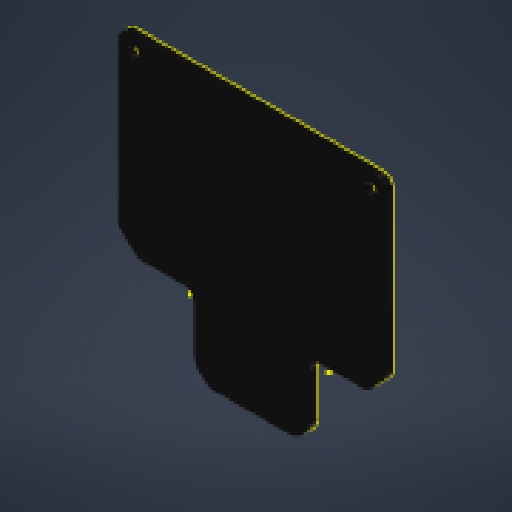
# Autodesk Inventor part: Motor Driver Board
Saved by Autodesk Inventor 2026.1 (Build 301233020, 233B)
## iProperties
Created: 2026-04-03
Part Number: Motor Driver Board
Material: Generic
Document SubType Name: Modeling
Designer: Bahaa
Density: 1 g/cm^3
Appearance: Glossy - Black
Mass: 8.08903 g
Surface Area: 86.5661 cm^2
Volume: 8.08903 cm^3
Author: Bahaa
Autodesk Inventor part; units mm, degrees
ref_plane "YZ Plane" through (0, 0, 0) normal (1, 0, 0) x (0, 1, 0)
ref_plane "XZ Plane" through (0, 0, 0) normal (0, 1, 0) x (-1, 0, 0)
ref_plane "XY Plane" through (0, 0, 0) normal (0, 0, 1) x (1, 0, 0)
sketch "Sketch1" plane through (0, 0, 0) normal (0, 1, 0) x (-1, 0, 0)
  line L0 (35, 25) -> (-35, 25)
  line L1 (-35, 25) -> (-35, -20)
  line L2 (-30, -25) -> (30, -25)
  line L3 (35, -20) -> (35, 25)
  line L4 (35, 25) -> (-35, -25) construction
  line L5 (-35, 25) -> (35, -25) construction
  line L6 (35, 25) -> (31, 25)
  line L7 (31, 25) -> (31, 21) construction
  line L8 (31, 21) -> (35, 21) construction
  line L9 (35, 21) -> (35, 25)
  line L10 (0, 25) -> (0, -25) construction
  circle A0 centre (31, 21) radius 1.6
  circle A1 centre (-31, 21) radius 1.6
  line L11 (15, -45) -> (-15, -45)
  line L12 (-15, -45) -> (-15, -5)
  line L13 (-15, -5) -> (15, -5)
  line L14 (15, -5) -> (15, -45)
  line L15 (15, -45) -> (-15, -5) construction
  line L16 (-15, -45) -> (15, -5) construction
  line L17 (27, 17) -> (35, 17) construction
  line L18 (35, 17) -> (35, 25) construction
  line L19 (35, 25) -> (27, 25) construction
  line L20 (27, 25) -> (27, 17) construction
  line L21 (27, 17) -> (35, 25) construction
  line L22 (35, 17) -> (27, 25) construction
  line L23 (-27, 17) -> (-35, 17) construction
  line L24 (-35, 17) -> (-35, 25) construction
  line L25 (-35, 25) -> (-27, 25) construction
  line L26 (-27, 25) -> (-27, 17) construction
  line L27 (-27, 17) -> (-35, 25) construction
  line L28 (-35, 17) -> (-27, 25) construction
  line L29 (35, -20) -> (30, -25)
  line L30 (-30, -25) -> (-35, -20)
  point P0 (0, 0)
  point P1 (15, -25)
  point P2 (-15, -25)
  dimension "d0" = 70
  dimension "d1" = 50
  dimension "d11" = 4
  dimension "d12" = 4
  dimension "d13" = 3.2
  dimension "d14" = 30
  dimension "d15" = 40
  dimension "d16" = 5
  dimension "d17" = 5
  dimension "d18" = 5
  dimension "d19" = 5
  constraints: 62 end point, 10 midpoint, 10 parallel, 5 horizontal, 5 perpendicular, 4 point on line, 2 centre point, 2 coincident, 1 symmetric about line, 1 other
  measures "d0" distance of L5.end L4.end
  measures "d1" distance of L4.end L0.end
  measures "d11" distance of L8.end L7.end
  measures "d12" distance of L7.end L6.end
  measures "d13" diameter of A0
  measures "d14" distance between parallel lines of L12 L14
  measures "d15" distance of L11.end L12.end
  measures "d16" distance of L3.start L5.end
  measures "d17" distance of L2.end L5.end
  measures "d18" distance of L2.start L4.end
  measures "d19" distance of L1.end L4.end
extrude "Extrusion1" add sketch "Sketch1" along normal blind 2
fillet "Fillet1" radius 3 8 edges at (-35, 1, 25) (35, 1, 25) (-15, 1, -25) (15, 1, -25) (30, 1, -25) (35, 1, -20) (-35, 1, -20) (-30, 1, -25)
chamfer "Chamfer1" distance 3.5 angle 45 2 edges at (-15, 1, -45) (15, 1, -45)
fillet "Fillet3" radius 4 4 edges at (15, 1, -41.5) (11.5, 1, -45) (-11.5, 1, -45) (-15, 1, -41.5)
sketch "Sketch2" plane through (0, 2, 0) normal (0, 1, 0) x (1, 0, 0)
  arc A0 (-9.8431, 45) -> (-12.6716, 43.8284) centre (-9.8431, 41) ccw projected
  line L0 (-9.8431, 45) -> (9.8431, 45) projected
  arc A1 (12.6716, 43.8284) -> (9.8431, 45) centre (9.8431, 41) ccw projected
  line L1 (12.6716, 43.8284) -> (13.8284, 42.6716) projected
  arc A2 (15, 39.8431) -> (13.8284, 42.6716) centre (11, 39.8431) ccw projected
  line L2 (15, 39.8431) -> (15, 28) projected
  arc A3 (15, 28) -> (18, 25) centre (18, 28) ccw projected
  line L3 (18, 25) -> (28.7574, 25) projected
  arc A4 (30.8787, 24.1213) -> (28.7574, 25) centre (28.7574, 22) ccw projected
  line L4 (30.8787, 24.1213) -> (34.1213, 20.8787) projected
  arc A5 (35, 18.7574) -> (34.1213, 20.8787) centre (32, 18.7574) ccw projected
  line L5 (35, 18.7574) -> (35, -22) projected
  arc A6 (32, -25) -> (35, -22) centre (32, -22) ccw projected
  line L6 (32, -25) -> (-32, -25) projected
  arc A7 (-35, -22) -> (-32, -25) centre (-32, -22) ccw projected
  line L7 (-35, -22) -> (-35, 18.7574) projected
  arc A8 (-34.1213, 20.8787) -> (-35, 18.7574) centre (-32, 18.7574) ccw projected
  line L8 (-34.1213, 20.8787) -> (-30.8787, 24.1213) projected
  arc A9 (-28.7574, 25) -> (-30.8787, 24.1213) centre (-28.7574, 22) ccw projected
  line L9 (-28.7574, 25) -> (-18, 25) projected
  arc A10 (-18, 25) -> (-15, 28) centre (-18, 28) ccw projected
  line L10 (-15, 28) -> (-15, 39.8431) projected
  arc A11 (-13.8284, 42.6716) -> (-15, 39.8431) centre (-11, 39.8431) ccw projected
  line L11 (-13.8284, 42.6716) -> (-12.6716, 43.8284) projected
  circle A12 centre (31, -21) radius 1.6 projected
  circle A13 centre (-31, -21) radius 1.6 projected
  line L12 (-13.31, 26.23) -> (-13.31, 38.93)
  line L13 (-13.31, 38.93) -> (-8.23, 38.93)
  line L14 (-8.23, 38.93) -> (-8.23, 26.23)
  line L15 (-8.23, 26.23) -> (-13.31, 26.23)
  line L16 (-12.14, 37.96) -> (-12.34, 37.96)
  line L17 (-12.34, 37.96) -> (-12.34, 37.36)
  line L18 (-12.34, 37.36) -> (-12.14, 37.36)
  line L19 (-12.14, 37.36) -> (-12.14, 37.41)
  line L20 (-12.14, 37.41) -> (-11.94, 37.41)
  line L21 (-11.94, 37.41) -> (-11.94, 37.36)
  line L22 (-11.94, 37.36) -> (-11.74, 37.36)
  line L23 (-11.74, 37.36) -> (-11.74, 37.96)
  line L24 (-11.74, 37.96) -> (-11.94, 37.96)
  line L25 (-11.94, 37.96) -> (-11.94, 37.91)
  line L26 (-11.94, 37.91) -> (-12.14, 37.91)
  line L27 (-12.14, 37.91) -> (-12.14, 37.96)
  line L28 (-12.14, 35.42) -> (-12.34, 35.42)
  line L29 (-12.34, 35.42) -> (-12.34, 34.82)
  line L30 (-12.34, 34.82) -> (-12.14, 34.82)
  line L31 (-12.14, 34.82) -> (-12.14, 34.87)
  line L32 (-12.14, 34.87) -> (-11.94, 34.87)
  line L33 (-11.94, 34.87) -> (-11.94, 34.82)
  line L34 (-11.94, 34.82) -> (-11.74, 34.82)
  line L35 (-11.74, 34.82) -> (-11.74, 35.42)
  line L36 (-11.74, 35.42) -> (-11.94, 35.42)
  line L37 (-11.94, 35.42) -> (-11.94, 35.37)
  line L38 (-11.94, 35.37) -> (-12.14, 35.37)
  line L39 (-12.14, 35.37) -> (-12.14, 35.42)
  line L40 (-12.14, 32.88) -> (-12.34, 32.88)
  line L41 (-12.34, 32.88) -> (-12.34, 32.28)
  line L42 (-12.34, 32.28) -> (-12.14, 32.28)
  line L43 (-12.14, 32.28) -> (-12.14, 32.33)
  line L44 (-12.14, 32.33) -> (-11.94, 32.33)
  line L45 (-11.94, 32.33) -> (-11.94, 32.28)
  line L46 (-11.94, 32.28) -> (-11.74, 32.28)
  line L47 (-11.74, 32.28) -> (-11.74, 32.88)
  line L48 (-11.74, 32.88) -> (-11.94, 32.88)
  line L49 (-11.94, 32.88) -> (-11.94, 32.83)
  line L50 (-11.94, 32.83) -> (-12.14, 32.83)
  line L51 (-12.14, 32.83) -> (-12.14, 32.88)
  line L52 (-12.14, 30.34) -> (-12.34, 30.34)
  line L53 (-12.34, 30.34) -> (-12.34, 29.74)
  line L54 (-12.34, 29.74) -> (-12.14, 29.74)
  line L55 (-12.14, 29.74) -> (-12.14, 29.79)
  line L56 (-12.14, 29.79) -> (-11.94, 29.79)
  line L57 (-11.94, 29.79) -> (-11.94, 29.74)
  line L58 (-11.94, 29.74) -> (-11.74, 29.74)
  line L59 (-11.74, 29.74) -> (-11.74, 30.34)
  line L60 (-11.74, 30.34) -> (-11.94, 30.34)
  line L61 (-11.94, 30.34) -> (-11.94, 30.29)
  line L62 (-11.94, 30.29) -> (-12.14, 30.29)
  line L63 (-12.14, 30.29) -> (-12.14, 30.34)
  line L64 (-12.14, 27.8) -> (-12.34, 27.8)
  line L65 (-12.34, 27.8) -> (-12.34, 27.2)
  line L66 (-12.34, 27.2) -> (-12.14, 27.2)
  line L67 (-12.14, 27.2) -> (-12.14, 27.25)
  line L68 (-12.14, 27.25) -> (-11.94, 27.25)
  line L69 (-11.94, 27.25) -> (-11.94, 27.2)
  line L70 (-11.94, 27.2) -> (-11.74, 27.2)
  line L71 (-11.74, 27.2) -> (-11.74, 27.8)
  line L72 (-11.74, 27.8) -> (-11.94, 27.8)
  line L73 (-11.94, 27.8) -> (-11.94, 27.75)
  line L74 (-11.94, 27.75) -> (-12.14, 27.75)
  line L75 (-12.14, 27.75) -> (-12.14, 27.8)
  line L76 (-9.4, 37.36) -> (-9.2, 37.36)
  line L77 (-9.2, 37.36) -> (-9.2, 37.96)
  line L78 (-9.2, 37.96) -> (-9.4, 37.96)
  line L79 (-9.4, 37.96) -> (-9.4, 37.91)
  line L80 (-9.4, 37.91) -> (-9.6, 37.91)
  line L81 (-9.6, 37.91) -> (-9.6, 37.96)
  line L82 (-9.6, 37.96) -> (-9.8, 37.96)
  line L83 (-9.8, 37.96) -> (-9.8, 37.36)
  line L84 (-9.8, 37.36) -> (-9.6, 37.36)
  line L85 (-9.6, 37.36) -> (-9.6, 37.41)
  line L86 (-9.6, 37.41) -> (-9.4, 37.41)
  line L87 (-9.4, 37.41) -> (-9.4, 37.36)
  line L88 (-9.4, 34.82) -> (-9.2, 34.82)
  line L89 (-9.2, 34.82) -> (-9.2, 35.42)
  line L90 (-9.2, 35.42) -> (-9.4, 35.42)
  line L91 (-9.4, 35.42) -> (-9.4, 35.37)
  line L92 (-9.4, 35.37) -> (-9.6, 35.37)
  line L93 (-9.6, 35.37) -> (-9.6, 35.42)
  line L94 (-9.6, 35.42) -> (-9.8, 35.42)
  line L95 (-9.8, 35.42) -> (-9.8, 34.82)
  line L96 (-9.8, 34.82) -> (-9.6, 34.82)
  line L97 (-9.6, 34.82) -> (-9.6, 34.87)
  line L98 (-9.6, 34.87) -> (-9.4, 34.87)
  line L99 (-9.4, 34.87) -> (-9.4, 34.82)
  line L100 (-9.4, 32.28) -> (-9.2, 32.28)
  line L101 (-9.2, 32.28) -> (-9.2, 32.88)
  line L102 (-9.2, 32.88) -> (-9.4, 32.88)
  line L103 (-9.4, 32.88) -> (-9.4, 32.83)
  line L104 (-9.4, 32.83) -> (-9.6, 32.83)
  line L105 (-9.6, 32.83) -> (-9.6, 32.88)
  line L106 (-9.6, 32.88) -> (-9.8, 32.88)
  line L107 (-9.8, 32.88) -> (-9.8, 32.28)
  line L108 (-9.8, 32.28) -> (-9.6, 32.28)
  line L109 (-9.6, 32.28) -> (-9.6, 32.33)
  line L110 (-9.6, 32.33) -> (-9.4, 32.33)
  line L111 (-9.4, 32.33) -> (-9.4, 32.28)
  line L112 (-9.4, 29.74) -> (-9.2, 29.74)
  line L113 (-9.2, 29.74) -> (-9.2, 30.34)
  line L114 (-9.2, 30.34) -> (-9.4, 30.34)
  line L115 (-9.4, 30.34) -> (-9.4, 30.29)
  line L116 (-9.4, 30.29) -> (-9.6, 30.29)
  line L117 (-9.6, 30.29) -> (-9.6, 30.34)
  line L118 (-9.6, 30.34) -> (-9.8, 30.34)
  line L119 (-9.8, 30.34) -> (-9.8, 29.74)
  line L120 (-9.8, 29.74) -> (-9.6, 29.74)
  line L121 (-9.6, 29.74) -> (-9.6, 29.79)
  line L122 (-9.6, 29.79) -> (-9.4, 29.79)
  line L123 (-9.4, 29.79) -> (-9.4, 29.74)
  line L124 (-9.4, 27.2) -> (-9.2, 27.2)
  line L125 (-9.2, 27.2) -> (-9.2, 27.8)
  line L126 (-9.2, 27.8) -> (-9.4, 27.8)
  line L127 (-9.4, 27.8) -> (-9.4, 27.75)
  line L128 (-9.4, 27.75) -> (-9.6, 27.75)
  line L129 (-9.6, 27.75) -> (-9.6, 27.8)
  line L130 (-9.6, 27.8) -> (-9.8, 27.8)
  line L131 (-9.8, 27.8) -> (-9.8, 27.2)
  line L132 (-9.8, 27.2) -> (-9.6, 27.2)
  line L133 (-9.6, 27.2) -> (-9.6, 27.25)
  line L134 (-9.6, 27.25) -> (-9.4, 27.25)
  line L135 (-9.4, 27.25) -> (-9.4, 27.2)
  line L136 (8.23, 26.23) -> (8.23, 38.93)
  line L137 (8.23, 38.93) -> (13.31, 38.93)
  line L138 (13.31, 38.93) -> (13.31, 26.23)
  line L139 (13.31, 26.23) -> (8.23, 26.23)
  line L140 (9.4, 37.96) -> (9.2, 37.96)
  line L141 (9.2, 37.96) -> (9.2, 37.36)
  line L142 (9.2, 37.36) -> (9.4, 37.36)
  line L143 (9.4, 37.36) -> (9.4, 37.41)
  line L144 (9.4, 37.41) -> (9.6, 37.41)
  line L145 (9.6, 37.41) -> (9.6, 37.36)
  line L146 (9.6, 37.36) -> (9.8, 37.36)
  line L147 (9.8, 37.36) -> (9.8, 37.96)
  line L148 (9.8, 37.96) -> (9.6, 37.96)
  line L149 (9.6, 37.96) -> (9.6, 37.91)
  line L150 (9.6, 37.91) -> (9.4, 37.91)
  line L151 (9.4, 37.91) -> (9.4, 37.96)
  line L152 (9.4, 35.42) -> (9.2, 35.42)
  line L153 (9.2, 35.42) -> (9.2, 34.82)
  line L154 (9.2, 34.82) -> (9.4, 34.82)
  line L155 (9.4, 34.82) -> (9.4, 34.87)
  line L156 (9.4, 34.87) -> (9.6, 34.87)
  line L157 (9.6, 34.87) -> (9.6, 34.82)
  line L158 (9.6, 34.82) -> (9.8, 34.82)
  line L159 (9.8, 34.82) -> (9.8, 35.42)
  line L160 (9.8, 35.42) -> (9.6, 35.42)
  line L161 (9.6, 35.42) -> (9.6, 35.37)
  line L162 (9.6, 35.37) -> (9.4, 35.37)
  line L163 (9.4, 35.37) -> (9.4, 35.42)
  line L164 (9.4, 32.88) -> (9.2, 32.88)
  line L165 (9.2, 32.88) -> (9.2, 32.28)
  line L166 (9.2, 32.28) -> (9.4, 32.28)
  line L167 (9.4, 32.28) -> (9.4, 32.33)
  line L168 (9.4, 32.33) -> (9.6, 32.33)
  line L169 (9.6, 32.33) -> (9.6, 32.28)
  line L170 (9.6, 32.28) -> (9.8, 32.28)
  line L171 (9.8, 32.28) -> (9.8, 32.88)
  line L172 (9.8, 32.88) -> (9.6, 32.88)
  line L173 (9.6, 32.88) -> (9.6, 32.83)
  line L174 (9.6, 32.83) -> (9.4, 32.83)
  line L175 (9.4, 32.83) -> (9.4, 32.88)
  line L176 (9.4, 30.34) -> (9.2, 30.34)
  line L177 (9.2, 30.34) -> (9.2, 29.74)
  line L178 (9.2, 29.74) -> (9.4, 29.74)
  line L179 (9.4, 29.74) -> (9.4, 29.79)
  line L180 (9.4, 29.79) -> (9.6, 29.79)
  line L181 (9.6, 29.79) -> (9.6, 29.74)
  line L182 (9.6, 29.74) -> (9.8, 29.74)
  line L183 (9.8, 29.74) -> (9.8, 30.34)
  line L184 (9.8, 30.34) -> (9.6, 30.34)
  line L185 (9.6, 30.34) -> (9.6, 30.29)
  line L186 (9.6, 30.29) -> (9.4, 30.29)
  line L187 (9.4, 30.29) -> (9.4, 30.34)
  line L188 (9.4, 27.8) -> (9.2, 27.8)
  line L189 (9.2, 27.8) -> (9.2, 27.2)
  line L190 (9.2, 27.2) -> (9.4, 27.2)
  line L191 (9.4, 27.2) -> (9.4, 27.25)
  line L192 (9.4, 27.25) -> (9.6, 27.25)
  line L193 (9.6, 27.25) -> (9.6, 27.2)
  line L194 (9.6, 27.2) -> (9.8, 27.2)
  line L195 (9.8, 27.2) -> (9.8, 27.8)
  line L196 (9.8, 27.8) -> (9.6, 27.8)
  line L197 (9.6, 27.8) -> (9.6, 27.75)
  line L198 (9.6, 27.75) -> (9.4, 27.75)
  line L199 (9.4, 27.75) -> (9.4, 27.8)
  line L200 (12.14, 37.36) -> (12.34, 37.36)
  line L201 (12.34, 37.36) -> (12.34, 37.96)
  line L202 (12.34, 37.96) -> (12.14, 37.96)
  line L203 (12.14, 37.96) -> (12.14, 37.91)
  line L204 (12.14, 37.91) -> (11.94, 37.91)
  line L205 (11.94, 37.91) -> (11.94, 37.96)
  line L206 (11.94, 37.96) -> (11.74, 37.96)
  line L207 (11.74, 37.96) -> (11.74, 37.36)
  line L208 (11.74, 37.36) -> (11.94, 37.36)
  line L209 (11.94, 37.36) -> (11.94, 37.41)
  line L210 (11.94, 37.41) -> (12.14, 37.41)
  line L211 (12.14, 37.41) -> (12.14, 37.36)
  line L212 (12.14, 34.82) -> (12.34, 34.82)
  line L213 (12.34, 34.82) -> (12.34, 35.42)
  line L214 (12.34, 35.42) -> (12.14, 35.42)
  line L215 (12.14, 35.42) -> (12.14, 35.37)
  line L216 (12.14, 35.37) -> (11.94, 35.37)
  line L217 (11.94, 35.37) -> (11.94, 35.42)
  line L218 (11.94, 35.42) -> (11.74, 35.42)
  line L219 (11.74, 35.42) -> (11.74, 34.82)
  line L220 (11.74, 34.82) -> (11.94, 34.82)
  line L221 (11.94, 34.82) -> (11.94, 34.87)
  line L222 (11.94, 34.87) -> (12.14, 34.87)
  line L223 (12.14, 34.87) -> (12.14, 34.82)
  line L224 (12.14, 32.28) -> (12.34, 32.28)
  line L225 (12.34, 32.28) -> (12.34, 32.88)
  line L226 (12.34, 32.88) -> (12.14, 32.88)
  line L227 (12.14, 32.88) -> (12.14, 32.83)
  line L228 (12.14, 32.83) -> (11.94, 32.83)
  line L229 (11.94, 32.83) -> (11.94, 32.88)
  line L230 (11.94, 32.88) -> (11.74, 32.88)
  line L231 (11.74, 32.88) -> (11.74, 32.28)
  line L232 (11.74, 32.28) -> (11.94, 32.28)
  line L233 (11.94, 32.28) -> (11.94, 32.33)
  line L234 (11.94, 32.33) -> (12.14, 32.33)
  line L235 (12.14, 32.33) -> (12.14, 32.28)
  line L236 (12.14, 29.74) -> (12.34, 29.74)
  line L237 (12.34, 29.74) -> (12.34, 30.34)
  line L238 (12.34, 30.34) -> (12.14, 30.34)
  line L239 (12.14, 30.34) -> (12.14, 30.29)
  line L240 (12.14, 30.29) -> (11.94, 30.29)
  line L241 (11.94, 30.29) -> (11.94, 30.34)
  line L242 (11.94, 30.34) -> (11.74, 30.34)
  line L243 (11.74, 30.34) -> (11.74, 29.74)
  line L244 (11.74, 29.74) -> (11.94, 29.74)
  line L245 (11.94, 29.74) -> (11.94, 29.79)
  line L246 (11.94, 29.79) -> (12.14, 29.79)
  line L247 (12.14, 29.79) -> (12.14, 29.74)
  line L248 (12.14, 27.2) -> (12.34, 27.2)
  line L249 (12.34, 27.2) -> (12.34, 27.8)
  line L250 (12.34, 27.8) -> (12.14, 27.8)
  line L251 (12.14, 27.8) -> (12.14, 27.75)
  line L252 (12.14, 27.75) -> (11.94, 27.75)
  line L253 (11.94, 27.75) -> (11.94, 27.8)
  line L254 (11.94, 27.8) -> (11.74, 27.8)
  line L255 (11.74, 27.8) -> (11.74, 27.2)
  line L256 (11.74, 27.2) -> (11.94, 27.2)
  line L257 (11.94, 27.2) -> (11.94, 27.25)
  line L258 (11.94, 27.25) -> (12.14, 27.25)
  line L259 (12.14, 27.25) -> (12.14, 27.2)
  point P0 (0, 0)
  constraints: 496 end point, 124 horizontal, 124 vertical, 248 other
sketch "Sketch3" plane through (0, 2, 0) normal (0, 1, 0) x (1, 0, 0)
  point P0 (0, 0)
equation "\"d17\" = d16"
equation "\"d18\" = d16"
equation "\"d19\" = d18"
body "Solid1"
